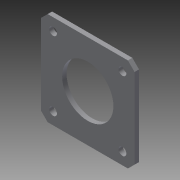
# Autodesk Inventor part: washer
Saved by Autodesk Inventor 2014 (Build 180170000, 170)
## iProperties
Created: 2014-11-20
Part Number: washer
Material: Generic
Document SubType Name: Modeling
Designer: KriMag
Density: 1 g/cm^3
Appearance: Default
Author: KriMag
Autodesk Inventor part; units mm, degrees
ref_plane "YZ Plane" through (0, 0, 0) normal (1, 0, 0) x (0, 1, 0)
ref_plane "XZ Plane" through (0, 0, 0) normal (0, 1, 0) x (-1, 0, 0)
ref_plane "XY Plane" through (0, 0, 0) normal (0, 0, 1) x (1, 0, 0)
sketch "Sketch1" plane through (0, 0, 0) normal (0, 1, 0) x (-1, 0, 0)
  line L0 (18, -21) -> (-18, -21)
  line L1 (-21, -18) -> (-21, 18)
  line L2 (-18, 21) -> (18, 21)
  line L3 (21, 18) -> (21, -18)
  line L4 (21, -21) -> (-21, 21) construction
  line L5 (-21, -21) -> (21, 21) construction
  line L6 (21, 18) -> (18, 21)
  line L7 (-21, -18) -> (-18, -21)
  line L8 (-18, 21) -> (-21, 18)
  line L9 (21, -18) -> (18, -21)
  line L10 (19.5, 19.5) -> (15.0999, 15.0999) construction
  circle A0 centre (15.5563, 15.5563) radius 1.75
  circle A1 centre (-15.5563, 15.5563) radius 1.75
  circle A2 centre (-15.5563, -15.5563) radius 1.75
  circle A3 centre (15.5563, -15.5563) radius 1.75
  circle A4 centre (0, 0) radius 11.5
  line L11 (-15.5563, 15.5563) -> (15.5563, -15.5563) construction
  dimension "d0" = 42
  dimension "d1" = 42
  dimension "d2" = 3
  dimension "d3" = 3
  dimension "d4" = 3
  dimension "d5" = 3
  dimension "d6" = 3
  dimension "d7" = 3
  dimension "d8" = 3
  dimension "d9" = 3
  dimension "d11" = 3.5
  dimension "d14" = 360
  dimension "d16" = 23
  dimension "d20" = 22
  constraints: 24 end point, 8 point on line, 5 centre point, 3 midpoint, 2 parallel, 1 coincident, 1 collinear, 1 horizontal, 1 perpendicular, 9 other
  measures "d0" distance of L4.end L5.end
  measures "d1" distance of L5.start L4.end
  measures "d2" distance of L3.start L5.end
  measures "d3" distance of L2.end L5.end
  measures "d4" distance of L1.start L5.start
  measures "d5" distance of L0.end L5.start
  measures "d6" distance of L2.start L4.end
  measures "d7" distance of L1.end L4.end
  measures "d8" distance of L3.end L4.start
  measures "d9" distance of L0.start L4.start
  measures "d11" diameter of A0
  measures "d16" diameter of A4
  measures "d20" distance of A0.centre point (0, 0)
extrude "Extrusion1" add sketch "Sketch1" along normal blind 2
equation "\"d3\" = d2"
equation "\"d5\" = d4"
equation "\"d7\" = d6"
equation "\"d9\" = d8"
body "Solid1"
